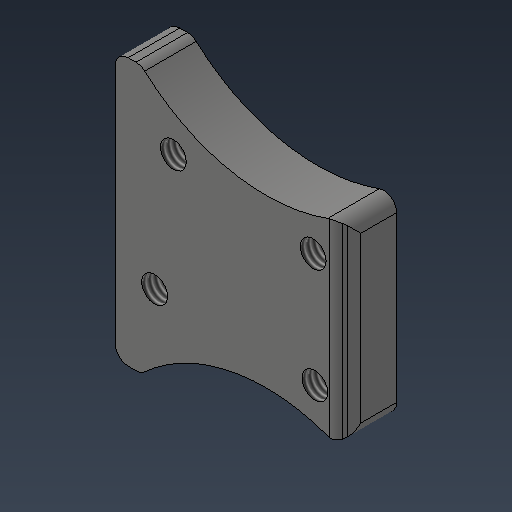
# Autodesk Inventor part: GearboxBearingHolderCover
Saved by Autodesk Inventor 2026.2 (Build 302298010, 298A)
## iProperties
Created: 2026-04-14
Part Number: GearboxBearingHolderCover
Material: Nylon 6/6
Document SubType Name: Modeling
Designer: szymo
Density: 1.13 g/cm^3
Appearance: Default(1)
Mass: 0.841862 g
Surface Area: 10.3759 cm^2
Volume: 0.74501 cm^3
Author: szymo
Autodesk Inventor part; units mm, degrees
ref_plane "YZ Plane" through (0, 0, 0) normal (1, 0, 0) x (0, 1, 0)
ref_plane "XZ Plane" through (0, 0, 0) normal (0, 1, 0) x (-1, 0, 0)
ref_plane "XY Plane" through (0, 0, 0) normal (0, 0, 1) x (1, 0, 0)
sketch "Sketch1" plane through (0, 0, 0) normal (0, 0, 1) x (1, 0, 0)
  line L0 (5, -24.795048) -> (3, -24.795048)
  line L1 (3, -24.795048) -> (3, -45.542024)
  line L2 (3, -45.542024) -> (5, -45.542024)
  circle A0 centre (14.7, -14.7) radius 14
  circle A1 centre (14.7, -55.637072) radius 14
  circle A2 centre (14.7, -14.7) radius 14.7 construction
  line L3 (0, -14.7) -> (0, -55.637072) construction
  circle A3 centre (14.7, -55.637072) radius 14.7 construction
  circle A4 centre (12.35, -35.272213) radius 5
  line L4 (20.85, -27.276864) -> (20.85, -43.060208)
  circle A5 centre (14.7, -14.7) radius 14.7 construction
  circle A6 centre (14.7, -14.7) radius 14
  circle A7 centre (14.7, -55.637072) radius 14.7 construction
  circle A8 centre (14.7, -55.637072) radius 14
  circle A9 centre (12.35, -35.272213) radius 3.2 construction
  circle A10 centre (12.35, -35.272213) radius 4.8 construction
  arc A11 (20.537456, -41.013777) -> (20.366204, -29.293879) centre (12.35, -35.272213) ccw
  line L5 (23.1, -65.837072) -> (23.1, -22.436494)
  arc A12 (20.537456, -41.013777) -> (19.161604, -37.17012) centre (18.490592, -39.578386) ccw
  line L6 (19.161604, -37.17012) -> (17.166531, -36.614236)
  arc A13 (17.166531, -36.614236) -> (17.125264, -33.790033) centre (12.35, -35.272213) ccw
  line L7 (17.125264, -33.790033) -> (19.103243, -33.176095)
  arc A14 (19.103243, -33.176095) -> (20.366204, -29.293879) centre (18.362153, -30.788463) ccw
  point P0 (0, 0)
  point P1 (20.85, -30.841023)
  point P2 (20.85, -39.496049)
  dimension "d0" = 3
  dimension "d2" = 3.5
  dimension "d5" = 10
  dimension "d6" = 2
  dimension "d7" = 2
  dimension "d22" = 20.74698
  constraints: 12 end point, 5 coincident, 4 point on circle, 4 vertical, 3 centre point, 2 concentric, 2 horizontal alignment, 2 perpendicular, 2 point on line, 1 horizontal, 8 other
  measures "d0" distance between parallel lines of L3 L1
  measures "d2" distance edge to line of A4 L4
  measures "d5" diameter of A4
  measures "d6" distance of L0.start L0.end
  measures "d7" distance of L1.end L2.end
  measures "d22" distance of L0.end L1.end
ref_plane "Work Plane1" through (5.561776, -42.060437, 3.6) normal (0, 0, 1) x (0.7075365, 0.7066768, 0)
ref_plane "Work Plane2" through (5.561776, -42.060437, 3.6) normal (0, 0, 1) x (0.7075365, 0.7066768, 0)
extrude "Extrusion1" add sketch "Sketch1" along normal up to surface (3.6 mm away) contours A0 L4 A11 A14 L7 A4 L6 A12 A1 L2 L1 L0 | L4 A14 A11 | A11 A12 L4 | L4 A12 L6 A4 L7 A14
sketch "Sketch2" plane through (3, -45.542024, 3.6) normal (0, 0, 1) x (1, 0, 0)
  circle A0 centre (9.35, 10.269811) radius 5
  line L0 (0, 0) -> (0, 20.746976)
  line L1 (2, 0) -> (0, 0)
  arc A1 (17.85, 2.481815) -> (2, 0) centre (11.7, -10.095048) ccw
  line L2 (17.85, 18.26516) -> (17.85, 2.481815)
  arc A2 (2, 20.746976) -> (17.85, 18.26516) centre (11.7, 30.842024) ccw
  line L3 (0, 20.746976) -> (2, 20.746976)
  line L4 (16.35, 16.396049) -> (16.35, 7.741023)
  point P0 (-3, 45.542024)
  constraints: 2 end point, 1 vertical
extrude "Extrusion2" add sketch "Sketch2" along normal blind 0.4 contours A0 | L0 L3 A2 L2 A1 L1
sketch "Sketch3" plane through (3, -45.542024, 0) normal (-1, 0, 0) x (0, 0, 1)
  line L0 (0, 20.746976) -> (4, 20.746976)
  line L1 (0, 20.746976) -> (0, 0)
  line L2 (0, 0) -> (4, 0)
  line L3 (4, 20.746976) -> (4, 0)
  line L4 (4, 10.373488) -> (0, 10.373488) construction
  circle A0 centre (2, 10.373488) radius 2
  line L5 (0, 15.269811) -> (0, 5.269811)
  point P0 (0, 45.542024)
  point P1 (2, 7.068536)
  constraints: 3 midpoint, 2 end point, 2 tangent, 1 centre point
hole "Hole1" at (3, -35.168536, 2) direction (1, 0, 0) diameter 2.013 depth 7 thread size "M2.5x0.45" class "6H" standard "ISO Metric profile"
chamfer "Chamfer2" distance 0.8 angle 45 1 edges at (20.85, -35.1685, 4) measured on face at (20.85, -35.1685, 3.5)
fillet "Fillet4" radius 1 8 edges at (20.85, -43.0602, 1.6) (20.85, -27.2769, 1.6) (5, -24.795, 2) (5, -45.542, 2) (3, -45.542, 2) (3, -24.795, 2) (20.85, -35.1685, 3.2) (20.05, -35.1685, 4)
sketch "Sketch5" plane through (0, 0, 0) normal (0, 0, -1) x (-1, 0, 0)
  arc A0 (-19.161604, -37.17012) -> (-16.455005, -41.029724) centre (-18.490592, -39.578386) ccw
  line L0 (-16.455005, -41.029724) -> (-15.252677, -39.343388)
  arc A1 (-17.166531, -36.614236) -> (-15.252677, -39.343388) centre (-12.35, -35.272213) ccw
  line L1 (-17.166531, -36.614236) -> (-19.161604, -37.17012)
  circle A2 centre (-18.490592, -39.578386) radius 1.35
  arc A3 (-16.28503, -29.39722) -> (-19.103243, -33.176095) centre (-18.362153, -30.788463) ccw
  line L2 (-19.103243, -33.176095) -> (-17.125264, -33.790033)
  arc A4 (-15.132486, -31.117965) -> (-17.125264, -33.790033) centre (-12.35, -35.272213) ccw
  line L3 (-15.132486, -31.117965) -> (-16.28503, -29.39722)
  circle A5 centre (-18.362153, -30.788463) radius 1.35
  arc A6 (-6.24345, -31.707098) -> (-9.841276, -28.661138) centre (-7.503908, -29.548106) ccw
  line L4 (-9.841276, -28.661138) -> (-10.576064, -30.597477)
  arc A7 (-8.032017, -32.751296) -> (-10.576064, -30.597477) centre (-12.35, -35.272213) ccw
  line L5 (-8.032017, -32.751296) -> (-6.24345, -31.707098)
  circle A8 centre (-7.503908, -29.548106) radius 1.35
  arc A9 (-8.029001, -40.869441) -> (-5.163114, -37.004369) centre (-6.050082, -39.341737) ccw
  line L6 (-5.163114, -37.004369) -> (-7.426827, -36.145351)
  arc A10 (-9.294592, -39.230051) -> (-7.426827, -36.145351) centre (-12.35, -35.272213) ccw
  line L7 (-9.294592, -39.230051) -> (-8.029001, -40.869441)
  circle A11 centre (-6.050082, -39.341737) radius 1.35
  point P0 (0, 0)
hole "Hole2" at (18.490592, -39.578386, 0) at (18.362153, -30.788463, 0) at (7.503908, -29.548106, 0) at (6.050082, -39.341737, 0) direction (0, 0, 1) diameter 2.013 end through all thread size "M2.5x0.45" class "6H" standard "ISO Metric profile"
equation "\"d7\" = d6"
body "Solid1"
